Autodesk Fusion 360 part; units mm, degrees
(part 5 of 7)
  spline S12 degree 5 poles (-11.7607, -34.2754) (-11.7671, -34.2886) (-11.7798, -34.3151) (-11.7979, -34.3554) (-11.8201, -34.4098) (-11.8455, -34.4789) (-11.8692, -34.5488) (-11.8917, -34.619) (-11.9136, -34.6896) (-11.9352, -34.7603) (-11.9563, -34.8311) (-11.9769, -34.9022) (-11.9967, -34.9736) (-12.0157, -35.0453) (-12.0338, -35.1173) (-12.0511, -35.1896) (-12.0678, -35.2622) (-12.0838, -35.3349) (-12.0994, -35.4079) (-12.1145, -35.481) (-12.1291, -35.5542) (-12.1432, -35.6277) (-12.1568, -35.7013) (-12.1698, -35.775) (-12.1823, -35.849) (-12.1944, -35.9231) (-12.2059, -35.9974) (-12.2169, -36.0718) (-12.2275, -36.1463) (-12.2377, -36.221) (-12.2474, -36.2958) (-12.2567, -36.3708) (-12.2656, -36.4458) (-12.274, -36.521) (-12.282, -36.5963) (-12.2896, -36.6717) (-12.2968, -36.7473) (-12.3036, -36.8229) (-12.3099, -36.8987) (-12.3159, -36.9745) (-12.3215, -37.0505) (-12.3267, -37.1265) (-12.3315, -37.2027) (-12.336, -37.2789) (-12.34, -37.3553) (-12.3437, -37.4317) (-12.347, -37.5082) (-12.35, -37.5848) (-12.3525, -37.6615) (-12.3548, -37.7383) (-12.3566, -37.8151) (-12.3581, -37.892) (-12.3593, -37.969) (-12.3601, -38.0461) (-12.3606, -38.1232) (-12.3607, -38.2004) (-12.3605, -38.2777) (-12.3599, -38.3551) (-12.359, -38.4325) (-12.3578, -38.51) (-12.3562, -38.5875) (-12.3543, -38.6651) (-12.3521, -38.7428) (-12.3495, -38.8205) (-12.3467, -38.8983) (-12.3435, -38.9761) (-12.34, -39.054) (-12.3361, -39.132) (-12.332, -39.21) (-12.3275, -39.288) (-12.3227, -39.3661) (-12.3186, -39.4286) (-12.3154, -39.4756) (-12.3132, -39.5068) (-12.3121, -39.5225) knots 0 0 0 0 0 0 0.01428571 0.02857143 0.04285714 0.05714286 0.07142857 0.08571429 0.1 0.11428571 0.12857143 0.14285714 0.15714286 0.17142857 0.18571429 0.2 0.21428571 0.22857143 0.24285714 0.25714286 0.27142857 0.28571429 0.3 0.31428571 0.32857143 0.34285714 0.35714286 0.37142857 0.38571429 0.4 0.41428571 0.42857143 0.44285714 0.45714286 0.47142857 0.48571429 0.5 0.51428571 0.52857143 0.54285714 0.55714286 0.57142857 0.58571429 0.6 0.61428571 0.62857143 0.64285714 0.65714286 0.67142857 0.68571429 0.7 0.71428571 0.72857143 0.74285714 0.75714286 0.77142857 0.78571429 0.8 0.81428571 0.82857143 0.84285714 0.85714286 0.87142857 0.88571429 0.9 0.91428571 0.92857143 0.94285714 0.95714286 0.97142857 0.98571429 1 1 1 1 1 1
  arc A27 (-12.3121, -39.5225) -> (-10.5685, -40.2447) centre (5.08, 0) ccw
  spline S13 degree 5 poles (-10.5685, -40.2447) (-10.5567, -40.2344) (-10.533, -40.2139) (-10.4976, -40.183) (-10.4505, -40.1416) (-10.3919, -40.0898) (-10.3335, -40.0378) (-10.2754, -39.9855) (-10.2176, -39.9331) (-10.16, -39.8806) (-10.1027, -39.8278) (-10.0457, -39.7748) (-9.9889, -39.7217) (-9.9325, -39.6683) (-9.8762, -39.6148) (-9.8203, -39.561) (-9.7646, -39.5071) (-9.7093, -39.453) (-9.6542, -39.3987) (-9.5994, -39.3442) (-9.5448, -39.2895) (-9.4906, -39.2347) (-9.4367, -39.1796) (-9.3831, -39.1243) (-9.3298, -39.0689) (-9.2767, -39.0132) (-9.224, -38.9574) (-9.1716, -38.9013) (-9.1196, -38.8451) (-9.0678, -38.7886) (-9.0164, -38.732) (-8.9652, -38.6751) (-8.9145, -38.6181) (-8.864, -38.5608) (-8.8139, -38.5034) (-8.7642, -38.4457) (-8.7148, -38.3878) (-8.6657, -38.3298) (-8.617, -38.2715) (-8.5687, -38.213) (-8.5207, -38.1543) (-8.4731, -38.0954) (-8.4259, -38.0363) (-8.3791, -37.9769) (-8.3327, -37.9174) (-8.2867, -37.8576) (-8.2411, -37.7976) (-8.1958, -37.7374) (-8.151, -37.6769) (-8.1067, -37.6163) (-8.0627, -37.5554) (-8.0193, -37.4942) (-7.9764, -37.4329) (-7.9339, -37.3712) (-7.892, -37.3093) (-7.8505, -37.2472) (-7.8095, -37.1848) (-7.7689, -37.1222) (-7.7288, -37.0594) (-7.6893, -36.9964) (-7.6504, -36.933) (-7.6122, -36.8692) (-7.575, -36.8051) (-7.5385, -36.7406) (-7.5028, -36.6758) (-7.4677, -36.6108) (-7.4329, -36.5456) (-7.3986, -36.4802) (-7.3648, -36.4145) (-7.3321, -36.3484) (-7.3012, -36.2816) (-7.2785, -36.2274) (-7.2628, -36.1862) (-7.253, -36.1584) (-7.2482, -36.1445) knots -1 -1 -1 -1 -1 -1 -0.98571429 -0.97142857 -0.95714286 -0.94285714 -0.92857143 -0.91428571 -0.9 -0.88571429 -0.87142857 -0.85714286 -0.84285714 -0.82857143 -0.81428571 -0.8 -0.78571429 -0.77142857 -0.75714286 -0.74285714 -0.72857143 -0.71428571 -0.7 -0.68571429 -0.67142857 -0.65714286 -0.64285714 -0.62857143 -0.61428571 -0.6 -0.58571429 -0.57142857 -0.55714286 -0.54285714 -0.52857143 -0.51428571 -0.5 -0.48571429 -0.47142857 -0.45714286 -0.44285714 -0.42857143 -0.41428571 -0.4 -0.38571429 -0.37142857 -0.35714286 -0.34285714 -0.32857143 -0.31428571 -0.3 -0.28571429 -0.27142857 -0.25714286 -0.24285714 -0.22857143 -0.21428571 -0.2 -0.18571429 -0.17142857 -0.15714286 -0.14285714 -0.12857143 -0.11428571 -0.1 -0.08571429 -0.07142857 -0.05714286 -0.04285714 -0.02857143 -0.01428571 0 0 0 0 0 0
  line L13 (-7.2482, -36.1445) -> (-7.1541, -35.8689)
  arc A28 (-6.7537, -35.6701) -> (-7.1541, -35.8689) centre (-6.8537, -35.9715) ccw
  arc A29 (-6.7537, -35.6701) -> (-4.8979, -36.2331) centre (5.08, 0) ccw
  arc A30 (-4.6754, -36.6208) -> (-4.8979, -36.2331) centre (-4.9822, -36.5392) ccw
  line L14 (-4.6754, -36.6208) -> (-4.7503, -36.9022)
  spline S14 degree 5 poles (-4.7503, -36.9022) (-4.7541, -36.9164) (-4.7613, -36.945) (-4.7712, -36.988) (-4.7824, -37.0457) (-4.7938, -37.1184) (-4.8034, -37.1915) (-4.8117, -37.2649) (-4.8195, -37.3383) (-4.8269, -37.4119) (-4.8338, -37.4855) (-4.8401, -37.5592) (-4.8456, -37.6331) (-4.8502, -37.7071) (-4.854, -37.7813) (-4.8568, -37.8556) (-4.859, -37.93) (-4.8605, -38.0045) (-4.8616, -38.0791) (-4.8621, -38.1537) (-4.8621, -38.2284) (-4.8616, -38.3032) (-4.8606, -38.378) (-4.859, -38.4529) (-4.8569, -38.5279) (-4.8542, -38.6029) (-4.851, -38.678) (-4.8473, -38.7531) (-4.8432, -38.8283) (-4.8386, -38.9036) (-4.8335, -38.9788) (-4.828, -39.0541) (-4.8221, -39.1295) (-4.8157, -39.2049) (-4.8088, -39.2803) (-4.8016, -39.3558) (-4.7939, -39.4312) (-4.7857, -39.5068) (-4.7772, -39.5823) (-4.7683, -39.6579) (-4.7589, -39.7334) (-4.7492, -39.809) (-4.7391, -39.8847) (-4.7286, -39.9603) (-4.7176, -40.036) (-4.7063, -40.1116) (-4.6947, -40.1873) (-4.6826, -40.263) (-4.6702, -40.3388) (-4.6574, -40.4145) (-4.6442, -40.4902) (-4.6307, -40.5659) (-4.6168, -40.6417) (-4.6026, -40.7174) (-4.588, -40.7932) (-4.573, -40.8689) (-4.5577, -40.9447) (-4.5421, -41.0205) (-4.5261, -41.0962) (-4.5098, -41.172) (-4.4931, -41.2477) (-4.4761, -41.3235) (-4.4588, -41.3992) (-4.4411, -41.4749) (-4.4231, -41.5507) (-4.4048, -41.6264) (-4.3862, -41.7021) (-4.3672, -41.7778) (-4.3479, -41.8535) (-4.3283, -41.9292) (-4.3084, -42.0048) (-4.2922, -42.0653) (-4.2799, -42.1107) (-4.2716, -42.141) (-4.2675, -42.1561) knots 0 0 0 0 0 0 0.01428571 0.02857143 0.04285714 0.05714286 0.07142857 0.08571429 0.1 0.11428571 0.12857143 0.14285714 0.15714286 0.17142857 0.18571429 0.2 0.21428571 0.22857143 0.24285714 0.25714286 0.27142857 0.28571429 0.3 0.31428571 0.32857143 0.34285714 0.35714286 0.37142857 0.38571429 0.4 0.41428571 0.42857143 0.44285714 0.45714286 0.47142857 0.48571429 0.5 0.51428571 0.52857143 0.54285714 0.55714286 0.57142857 0.58571429 0.6 0.61428571 0.62857143 0.64285714 0.65714286 0.67142857 0.68571429 0.7 0.71428571 0.72857143 0.74285714 0.75714286 0.77142857 0.78571429 0.8 0.81428571 0.82857143 0.84285714 0.85714286 0.87142857 0.88571429 0.9 0.91428571 0.92857143 0.94285714 0.95714286 0.97142857 0.98571429 1 1 1 1 1 1
  arc A31 (-4.2675, -42.1561) -> (-2.4165, -42.5243) centre (5.08, 0) ccw
  spline S15 degree 5 poles (-2.4165, -42.5243) (-2.4069, -42.5119) (-2.3877, -42.4871) (-2.3589, -42.4499) (-2.3208, -42.4002) (-2.2735, -42.3379) (-2.2264, -42.2755) (-2.1796, -42.2129) (-2.1331, -42.1503) (-2.0869, -42.0874) (-2.041, -42.0245) (-1.9954, -41.9614) (-1.9501, -41.8982) (-1.9051, -41.8349) (-1.8604, -41.7714) (-1.816, -41.7078) (-1.7719, -41.6441) (-1.7282, -41.5802) (-1.6847, -41.5162) (-1.6416, -41.452) (-1.5988, -41.3878) (-1.5564, -41.3234) (-1.5142, -41.2588) (-1.4724, -41.1942) (-1.4309, -41.1294) (-1.3898, -41.0644) (-1.349, -40.9994) (-1.3085, -40.9342) (-1.2684, -40.8689) (-1.2287, -40.8034) (-1.1893, -40.7378) (-1.1502, -40.6721) (-1.1116, -40.6062) (-1.0733, -40.5402) (-1.0353, -40.4741) (-0.9978, -40.4079) (-0.9606, -40.3415) (-0.9238, -40.2749) (-0.8874, -40.2083) (-0.8514, -40.1415) (-0.8158, -40.0746) (-0.7806, -40.0075) (-0.7459, -39.9403) (-0.7116, -39.873) (-0.6777, -39.8055) (-0.6442, -39.7379) (-0.6112, -39.6701) (-0.5786, -39.6023) (-0.5464, -39.5342) (-0.5147, -39.4661) (-0.4835, -39.3978) (-0.4528, -39.3293) (-0.4227, -39.2608) (-0.3931, -39.192) (-0.364, -39.1231) (-0.3355, -39.0541) (-0.3074, -38.9849) (-0.2798, -38.9156) (-0.2528, -38.8462) (-0.2263, -38.7766) (-0.2005, -38.7069) (-0.1755, -38.6369) (-0.1515, -38.5668) (-0.1283, -38.4964) (-0.106, -38.4259) (-0.0842, -38.3553) (-0.0628, -38.2845) (-0.0419, -38.2136) (-0.0216, -38.1427) (-0.0024, -38.0715) (0.0149, -37.9999) (0.0266, -37.9423) (0.0339, -37.8988) (0.0382, -37.8697) (0.0401, -37.8551) knots -1 -1 -1 -1 -1 -1 -0.98571429 -0.97142857 -0.95714286 -0.94285714 -0.92857143 -0.91428571 -0.9 -0.88571429 -0.87142857 -0.85714286 -0.84285714 -0.82857143 -0.81428571 -0.8 -0.78571429 -0.77142857 -0.75714286 -0.74285714 -0.72857143 -0.71428571 -0.7 -0.68571429 -0.67142857 -0.65714286 -0.64285714 -0.62857143 -0.61428571 -0.6 -0.58571429 -0.57142857 -0.55714286 -0.54285714 -0.52857143 -0.51428571 -0.5 -0.48571429 -0.47142857 -0.45714286 -0.44285714 -0.42857143 -0.41428571 -0.4 -0.38571429 -0.37142857 -0.35714286 -0.34285714 -0.32857143 -0.31428571 -0.3 -0.28571429 -0.27142857 -0.25714286 -0.24285714 -0.22857143 -0.21428571 -0.2 -0.18571429 -0.17142857 -0.15714286 -0.14285714 -0.12857143 -0.11428571 -0.1 -0.08571429 -0.07142857 -0.05714286 -0.04285714 -0.02857143 -0.01428571 0 0 0 0 0 0
  line L15 (0.0401, -37.8551) -> (0.0786, -37.5665)
  arc A32 (0.4326, -37.2934) -> (0.0786, -37.5665) centre (0.3933, -37.6084) ccw
  arc A33 (0.4326, -37.2934) -> (2.3625, -37.4835) centre (5.08, 0) ccw
  arc A34 (2.6564, -37.8204) -> (2.3625, -37.4835) centre (2.3396, -37.8001) ccw
  line L16 (2.6564, -37.8204) -> (2.6379, -38.1109)
  spline S16 degree 5 poles (2.6379, -38.1109) (2.6369, -38.1256) (2.6354, -38.155) (2.6341, -38.1991) (2.6344, -38.2579) (2.6374, -38.3315) (2.6423, -38.405) (2.6483, -38.4786) (2.6551, -38.5522) (2.6622, -38.6257) (2.6698, -38.6993) (2.678, -38.7728) (2.687, -38.8464) (2.6969, -38.9198) (2.7077, -38.9933) (2.7194, -39.0668) (2.7318, -39.1402) (2.7448, -39.2135) (2.7583, -39.2869) (2.7724, -39.3602) (2.7869, -39.4335) (2.802, -39.5067) (2.8176, -39.5799) (2.8337, -39.653) (2.8505, -39.7262) (2.8678, -39.7992) (2.8855, -39.8723) (2.9038, -39.9452) (2.9225, -40.0182) (2.9417, -40.0911) (2.9614, -40.1639) (2.9814, -40.2367) (3.002, -40.3094) (3.023, -40.3821) (3.0444, -40.4548) (3.0662, -40.5273) (3.0885, -40.5999) (3.1112, -40.6724) (3.1343, -40.7448) (3.1578, -40.8171) (3.1817, -40.8895) (3.206, -40.9617) (3.2307, -41.0339) (3.2558, -41.106) (3.2813, -41.1781) (3.3071, -41.2501) (3.3333, -41.3221) (3.3599, -41.394) (3.3869, -41.4658) (3.4142, -41.5376) (3.4419, -41.6093) (3.4699, -41.6809) (3.4983, -41.7525) (3.527, -41.824) (3.5561, -41.8955) (3.5856, -41.9669) (3.6154, -42.0382) (3.6455, -42.1094) (3.6759, -42.1806) (3.7067, -42.2517) (3.7378, -42.3228) (3.7693, -42.3938) (3.8011, -42.4647) (3.8332, -42.5355) (3.8656, -42.6063) (3.8983, -42.6769) (3.9314, -42.7476) (3.9648, -42.8181) (3.9985, -42.8886) (4.0325, -42.959) (4.0668, -43.0293) (4.0944, -43.0855) (4.1154, -43.1276) (4.1294, -43.1557) (4.1364, -43.1697) knots 0 0 0 0 0 0 0.01428571 0.02857143 0.04285714 0.05714286 0.07142857 0.08571429 0.1 0.11428571 0.12857143 0.14285714 0.15714286 0.17142857 0.18571429 0.2 0.21428571 0.22857143 0.24285714 0.25714286 0.27142857 0.28571429 0.3 0.31428571 0.32857143 0.34285714 0.35714286 0.37142857 0.38571429 0.4 0.41428571 0.42857143 0.44285714 0.45714286 0.47142857 0.48571429 0.5 0.51428571 0.52857143 0.54285714 0.55714286 0.57142857 0.58571429 0.6 0.61428571 0.62857143 0.64285714 0.65714286 0.67142857 0.68571429 0.7 0.71428571 0.72857143 0.74285714 0.75714286 0.77142857 0.78571429 0.8 0.81428571 0.82857143 0.84285714 0.85714286 0.87142857 0.88571429 0.9 0.91428571 0.92857143 0.94285714 0.95714286 0.97142857 0.98571429 1 1 1 1 1 1
  arc A35 (4.1364, -43.1697) -> (6.0236, -43.1697) centre (5.08, 0) ccw
  spline S17 degree 5 poles (6.0236, -43.1697) (6.0306, -43.1557) (6.0446, -43.1276) (6.0656, -43.0855) (6.0932, -43.0293) (6.1275, -42.959) (6.1615, -42.8886) (6.1952, -42.8181) (6.2286, -42.7476) (6.2617, -42.6769) (6.2944, -42.6063) (6.3268, -42.5355) (6.3589, -42.4647) (6.3907, -42.3938) (6.4222, -42.3228) (6.4533, -42.2517) (6.4841, -42.1806) (6.5145, -42.1094) (6.5446, -42.0382) (6.5744, -41.9669) (6.6039, -41.8955) (6.633, -41.824) (6.6617, -41.7525) (6.6901, -41.6809) (6.7181, -41.6093) (6.7458, -41.5376) (6.7731, -41.4658) (6.8001, -41.394) (6.8267, -41.3221) (6.8529, -41.2501) (6.8787, -41.1781) (6.9042, -41.106) (6.9293, -41.0339) (6.954, -40.9617) (6.9783, -40.8895) (7.0022, -40.8171) (7.0257, -40.7448) (7.0488, -40.6724) (7.0715, -40.5999) (7.0938, -40.5273) (7.1156, -40.4548) (7.137, -40.3821) (7.158, -40.3094) (7.1786, -40.2367) (7.1986, -40.1639) (7.2183, -40.0911) (7.2375, -40.0182) (7.2562, -39.9452) (7.2745, -39.8723) (7.2922, -39.7992) (7.3095, -39.7262) (7.3263, -39.653) (7.3424, -39.5799) (7.358, -39.5067) (7.3731, -39.4335) (7.3876, -39.3602) (7.4017, -39.2869) (7.4152, -39.2135) (7.4282, -39.1402) (7.4406, -39.0668) (7.4523, -38.9933) (7.4631, -38.9198) (7.473, -38.8464) (7.482, -38.7728) (7.4902, -38.6993) (7.4978, -38.6257) (7.5049, -38.5522) (7.5117, -38.4786) (7.5177, -38.405) (7.5226, -38.3315) (7.5256, -38.2579) (7.5259, -38.1991) (7.5246, -38.155) (7.5231, -38.1256) (7.5221, -38.1109) knots -1 -1 -1 -1 -1 -1 -0.98571429 -0.97142857 -0.95714286 -0.94285714 -0.92857143 -0.91428571 -0.9 -0.88571429 -0.87142857 -0.85714286 -0.84285714 -0.82857143 -0.81428571 -0.8 -0.78571429 -0.77142857 -0.75714286 -0.74285714 -0.72857143 -0.71428571 -0.7 -0.68571429 -0.67142857 -0.65714286 -0.64285714 -0.62857143 -0.61428571 -0.6 -0.58571429 -0.57142857 -0.55714286 -0.54285714 -0.52857143 -0.51428571 -0.5 -0.48571429 -0.47142857 -0.45714286 -0.44285714 -0.42857143 -0.41428571 -0.4 -0.38571429 -0.37142857 -0.35714286 -0.34285714 -0.32857143 -0.31428571 -0.3 -0.28571429 -0.27142857 -0.25714286 -0.24285714 -0.22857143 -0.21428571 -0.2 -0.18571429 -0.17142857 -0.15714286 -0.14285714 -0.12857143 -0.11428571 -0.1 -0.08571429 -0.07142857 -0.05714286 -0.04285714 -0.02857143 -0.01428571 0 0 0 0 0 0
  line L17 (7.5221, -38.1109) -> (7.5036, -37.8204)
  arc A36 (7.7975, -37.4835) -> (7.5036, -37.8204) centre (7.8204, -37.8001) ccw
  arc A37 (7.7975, -37.4835) -> (9.7274, -37.2934) centre (5.08, 0) ccw
  arc A38 (10.0814, -37.5665) -> (9.7274, -37.2934) centre (9.7667, -37.6084) ccw
  line L18 (10.0814, -37.5665) -> (10.1199, -37.8551)
  spline S18 degree 5 poles (10.1199, -37.8551) (10.1218, -37.8697) (10.1261, -37.8988) (10.1334, -37.9423) (10.1451, -37.9999) (10.1624, -38.0715) (10.1816, -38.1427) (10.2019, -38.2136) (10.2228, -38.2845) (10.2442, -38.3553) (10.266, -38.4259) (10.2883, -38.4964) (10.3115, -38.5668) (10.3355, -38.6369) (10.3605, -38.7069) (10.3863, -38.7766) (10.4128, -38.8462) (10.4398, -38.9156) (10.4674, -38.9849) (10.4955, -39.0541) (10.524, -39.1231) (10.5531, -39.192) (10.5827, -39.2608) (10.6128, -39.3293) (10.6435, -39.3978) (10.6747, -39.4661) (10.7064, -39.5342) (10.7386, -39.6023) (10.7712, -39.6701) (10.8042, -39.7379) (10.8377, -39.8055) (10.8716, -39.873) (10.9059, -39.9403) (10.9406, -40.0075) (10.9758, -40.0746) (11.0114, -40.1415) (11.0474, -40.2083) (11.0838, -40.2749) (11.1206, -40.3415) (11.1578, -40.4079) (11.1953, -40.4741) (11.2333, -40.5402) (11.2716, -40.6062) (11.3102, -40.6721) (11.3493, -40.7378) (11.3887, -40.8034) (11.4284, -40.8689) (11.4685, -40.9342) (11.509, -40.9994) (11.5498, -41.0644) (11.5909, -41.1294) (11.6324, -41.1942) (11.6742, -41.2588) (11.7164, -41.3234) (11.7588, -41.3878) (11.8016, -41.452) (11.8447, -41.5162) (11.8882, -41.5802) (11.9319, -41.6441) (11.976, -41.7078) (12.0204, -41.7714) (12.0651, -41.8349) (12.1101, -41.8982) (12.1554, -41.9614) (12.201, -42.0245) (12.2469, -42.0874) (12.2931, -42.1503) (12.3396, -42.2129) (12.3864, -42.2755) (12.4335, -42.3379) (12.4808, -42.4002) (12.5189, -42.4499) (12.5477, -42.4871) (12.5669, -42.5119) (12.5765, -42.5243) knots 0 0 0 0 0 0 0.01428571 0.02857143 0.04285714 0.05714286 0.07142857 0.08571429 0.1 0.11428571 0.12857143 0.14285714 0.15714286 0.17142857 0.18571429 0.2 0.21428571 0.22857143 0.24285714 0.25714286 0.27142857 0.28571429 0.3 0.31428571 0.32857143 0.34285714 0.35714286 0.37142857 0.38571429 0.4 0.41428571 0.42857143 0.44285714 0.45714286 0.47142857 0.48571429 0.5 0.51428571 0.52857143 0.54285714 0.55714286 0.57142857 0.58571429 0.6 0.61428571 0.62857143 0.64285714 0.65714286 0.67142857 0.68571429 0.7 0.71428571 0.72857143 0.74285714 0.75714286 0.77142857 0.78571429 0.8 0.81428571 0.82857143 0.84285714 0.85714286 0.87142857 0.88571429 0.9 0.91428571 0.92857143 0.94285714 0.95714286 0.97142857 0.98571429 1 1 1 1 1 1
  arc A39 (12.5765, -42.5243) -> (14.4275, -42.1561) centre (5.08, 0) ccw
  spline S19 degree 5 poles (14.4275, -42.1561) (14.4316, -42.141) (14.4399, -42.1107) (14.4522, -42.0653) (14.4684, -42.0048) (14.4883, -41.9292) (14.5079, -41.8535) (14.5272, -41.7778) (14.5462, -41.7021) (14.5648, -41.6264) (14.5831, -41.5507) (14.6011, -41.4749) (14.6188, -41.3992) (14.6361, -41.3235) (14.6531, -41.2477) (14.6698, -41.172) (14.6861, -41.0962) (14.7021, -41.0205) (14.7177, -40.9447) (14.733, -40.8689) (14.748, -40.7932) (14.7626, -40.7174) (14.7768, -40.6417) (14.7907, -40.5659) (14.8042, -40.4902) (14.8174, -40.4145) (14.8302, -40.3388) (14.8426, -40.263) (14.8547, -40.1873) (14.8663, -40.1116) (14.8776, -40.036) (14.8886, -39.9603) (14.8991, -39.8847) (14.9092, -39.809) (14.9189, -39.7334) (14.9283, -39.6579) (14.9372, -39.5823) (14.9457, -39.5068) (14.9539, -39.4312) (14.9616, -39.3558) (14.9688, -39.2803) (14.9757, -39.2049) (14.9821, -39.1295) (14.988, -39.0541) (14.9935, -38.9788) (14.9986, -38.9036) (15.0032, -38.8283) (15.0073, -38.7531) (15.011, -38.678) (15.0142, -38.6029) (15.0169, -38.5279) (15.019, -38.4529) (15.0206, -38.378) (15.0216, -38.3032) (15.0221, -38.2284) (15.0221, -38.1537) (15.0216, -38.0791) (15.0205, -38.0045) (15.019, -37.93) (15.0168, -37.8556) (15.014, -37.7813) (15.0102, -37.7071) (15.0056, -37.6331) (15.0001, -37.5592) (14.9938, -37.4855) (14.9869, -37.4119) (14.9795, -37.3383) (14.9717, -37.2649) (14.9634, -37.1915) (14.9538, -37.1184) (14.9424, -37.0457) (14.9312, -36.988) (14.9213, -36.945) (14.9141, -36.9164) (14.9103, -36.9022) knots -1 -1 -1 -1 -1 -1 -0.98571429 -0.97142857 -0.95714286 -0.94285714 -0.92857143 -0.91428571 -0.9 -0.88571429 -0.87142857 -0.85714286 -0.84285714 -0.82857143 -0.81428571 -0.8 -0.78571429 -0.77142857 -0.75714286 -0.74285714 -0.72857143 -0.71428571 -0.7 -0.68571429 -0.67142857 -0.65714286 -0.64285714 -0.62857143 -0.61428571 -0.6 -0.58571429 -0.57142857 -0.55714286 -0.54285714 -0.52857143 -0.51428571 -0.5 -0.48571429 -0.47142857 -0.45714286 -0.44285714 -0.42857143 -0.41428571 -0.4 -0.38571429 -0.37142857 -0.35714286 -0.34285714 -0.32857143 -0.31428571 -0.3 -0.28571429 -0.27142857 -0.25714286 -0.24285714 -0.22857143 -0.21428571 -0.2 -0.18571429 -0.17142857 -0.15714286 -0.14285714 -0.12857143 -0.11428571 -0.1 -0.08571429 -0.07142857 -0.05714286 -0.04285714 -0.02857143 -0.01428571 0 0 0 0 0 0
  line L19 (14.9103, -36.9022) -> (14.8354, -36.6208)
  arc A40 (15.0579, -36.2331) -> (14.8354, -36.6208) centre (15.1422, -36.5392) ccw
  arc A41 (15.0579, -36.2331) -> (16.9137, -35.6701) centre (5.08, 0) ccw
  arc A42 (17.3141, -35.8689) -> (16.9137, -35.6701) centre (17.0137, -35.9715) ccw
  line L20 (17.3141, -35.8689) -> (17.4082, -36.1445)
  spline S20 degree 5 poles (17.4082, -36.1445) (17.413, -36.1584) (17.4228, -36.1862) (17.4385, -36.2274) (17.4612, -36.2816) (17.4921, -36.3484) (17.5248, -36.4145) (17.5586, -36.4802) (17.5929, -36.5456) (17.6277, -36.6108) (17.6628, -36.6758) (17.6985, -36.7406) (17.735, -36.8051) (17.7722, -36.8692) (17.8104, -36.933) (17.8493, -36.9964) (17.8888, -37.0594) (17.9289, -37.1222) (17.9695, -37.1848) (18.0105, -37.2472) (18.052, -37.3093) (18.0939, -37.3712) (18.1364, -37.4329) (18.1793, -37.4942) (18.2227, -37.5554) (18.2667, -37.6163) (18.311, -37.6769) (18.3558, -37.7374) (18.4011, -37.7976) (18.4467, -37.8576) (18.4927, -37.9174) (18.5391, -37.9769) (18.5859, -38.0363) (18.6331, -38.0954) (18.6807, -38.1543) (18.7287, -38.213) (18.777, -38.2715) (18.8257, -38.3298) (18.8748, -38.3878) (18.9242, -38.4457) (18.9739, -38.5034) (19.024, -38.5608) (19.0745, -38.6181) (19.1252, -38.6751) (19.1764, -38.732) (19.2278, -38.7886) (19.2796, -38.8451) (19.3316, -38.9013) (19.384, -38.9574) (19.4367, -39.0132) (19.4898, -39.0689) (19.5431, -39.1243) (19.5967, -39.1796) (19.6506, -39.2347) (19.7048, -39.2895) (19.7594, -39.3442) (19.8142, -39.3987) (19.8693, -39.453) (19.9246, -39.5071) (19.9803, -39.561) (20.0362, -39.6148) (20.0925, -39.6683) (20.1489, -39.7217) (20.2057, -39.7748) (20.2627, -39.8278) (20.32, -39.8806) (20.3776, -39.9331) (20.4354, -39.9855) (20.4935, -40.0378) (20.5519, -40.0898) (20.6105, -40.1416) (20.6576, -40.183) (20.693, -40.2139) (20.7167, -40.2344) (20.7285, -40.2447) knots 0 0 0 0 0 0 0.01428571 0.02857143 0.04285714 0.05714286 0.07142857 0.08571429 0.1 0.11428571 0.12857143 0.14285714 0.15714286 0.17142857 0.18571429 0.2 0.21428571 0.22857143 0.24285714 0.25714286 0.27142857 0.28571429 0.3 0.31428571 0.32857143 0.34285714 0.35714286 0.37142857 0.38571429 0.4 0.41428571 0.42857143 0.44285714 0.45714286 0.47142857 0.48571429 0.5 0.51428571 0.52857143 0.54285714 0.55714286 0.57142857 0.58571429 0.6 0.61428571 0.62857143 0.64285714 0.65714286 0.67142857 0.68571429 0.7 0.71428571 0.72857143 0.74285714 0.75714286 0.77142857 0.78571429 0.8 0.81428571 0.82857143 0.84285714 0.85714286 0.87142857 0.88571429 0.9 0.91428571 0.92857143 0.94285714 0.95714286 0.97142857 0.98571429 1 1 1 1 1 1
  arc A43 (20.7285, -40.2447) -> (22.4721, -39.5225) centre (5.08, 0) ccw
  spline S21 degree 5 poles (22.4721, -39.5225) (22.4732, -39.5068) (22.4754, -39.4756) (22.4786, -39.4286) (22.4827, -39.3661) (22.4875, -39.288) (22.492, -39.21) (22.4961, -39.132) (22.5, -39.054) (22.5035, -38.9761) (22.5067, -38.8983) (22.5095, -38.8205) (22.5121, -38.7428) (22.5143, -38.6651) (22.5162, -38.5875) (22.5178, -38.51) (22.519, -38.4325) (22.5199, -38.3551) (22.5205, -38.2777) (22.5207, -38.2004) (22.5206, -38.1232) (22.5201, -38.0461) (22.5193, -37.969) (22.5181, -37.892) (22.5166, -37.8151) (22.5148, -37.7383) (22.5125, -37.6615) (22.51, -37.5848) (22.507, -37.5082) (22.5037, -37.4317) (22.5, -37.3553) (22.496, -37.2789) (22.4915, -37.2027) (22.4867, -37.1265) (22.4815, -37.0505) (22.4759, -36.9745) (22.4699, -36.8987) (22.4636, -36.8229) (22.4568, -36.7473) (22.4496, -36.6717) (22.442, -36.5963) (22.434, -36.521) (22.4256, -36.4458) (22.4167, -36.3708) (22.4074, -36.2958) (22.3977, -36.221) (22.3875, -36.1463) (22.3769, -36.0718) (22.3659, -35.9974) (22.3544, -35.9231) (22.3423, -35.849) (22.3298, -35.775) (22.3168, -35.7013) (22.3032, -35.6277) (22.2891, -35.5542) (22.2745, -35.481) (22.2594, -35.4079) (22.2438, -35.3349) (22.2278, -35.2622) (22.2111, -35.1896) (22.1938, -35.1173) (22.1757, -35.0453) (22.1567, -34.9736) (22.1369, -34.9022) (22.1163, -34.8311) (22.0952, -34.7603) (22.0736, -34.6896) (22.0517, -34.619) (22.0292, -34.5488) (22.0055, -34.4789) (21.9801, -34.4098) (21.9579, -34.3554) (21.9398, -34.3151) (21.9271, -34.2886) (21.9207, -34.2754) knots -1 -1 -1 -1 -1 -1 -0.98571429 -0.97142857 -0.95714286 -0.94285714 -0.92857143 -0.91428571 -0.9 -0.88571429 -0.87142857 -0.85714286 -0.84285714 -0.82857143 -0.81428571 -0.8 -0.78571429 -0.77142857 -0.75714286 -0.74285714 -0.72857143 -0.71428571 -0.7 -0.68571429 -0.67142857 -0.65714286 -0.64285714 -0.62857143 -0.61428571 -0.6 -0.58571429 -0.57142857 -0.55714286 -0.54285714 -0.52857143 -0.51428571 -0.5 -0.48571429 -0.47142857 -0.45714286 -0.44285714 -0.42857143 -0.41428571 -0.4 -0.38571429 -0.37142857 -0.35714286 -0.34285714 -0.32857143 -0.31428571 -0.3 -0.28571429 -0.27142857 -0.25714286 -0.24285714 -0.22857143 -0.21428571 -0.2 -0.18571429 -0.17142857 -0.15714286 -0.14285714 -0.12857143 -0.11428571 -0.1 -0.08571429 -0.07142857 -0.05714286 -0.04285714 -0.02857143 -0.01428571 0 0 0 0 0 0
  line L21 (21.9207, -34.2754) -> (21.7923, -34.014)
  arc A44 (21.9349, -33.5903) -> (21.7923, -34.014) centre (22.0773, -33.8741) ccw
  arc A45 (21.9349, -33.5903) -> (23.6452, -32.6761) centre (5.08, 0) ccw
  arc A46 (24.0768, -32.7929) -> (23.6452, -32.6761) centre (23.8021, -32.9522) ccw
  line L22 (24.0768, -32.7929) -> (24.2228, -33.0449)
  spline S22 degree 5 poles (24.2228, -33.0449) (24.2301, -33.0576) (24.2452, -33.0829) (24.2686, -33.1203) (24.3015, -33.169) (24.3449, -33.2285) (24.3898, -33.287) (24.4357, -33.3448) (24.4822, -33.4022) (24.529, -33.4594) (24.5762, -33.5163) (24.6238, -33.5729) (24.6721, -33.6291) (24.7212, -33.6847) (24.771, -33.7397) (24.8215, -33.7943) (24.8726, -33.8485) (24.9242, -33.9022) (24.9762, -33.9557) (25.0286, -34.0089) (25.0814, -34.0617) (25.1346, -34.1142) (25.1883, -34.1664) (25.2424, -34.2183) (25.2969, -34.2698) (25.3519, -34.3209) (25.4072, -34.3717) (25.463, -34.4223) (25.519, -34.4725) (25.5755, -34.5225) (25.6323, -34.5721) (25.6894, -34.6215) (25.7469, -34.6706) (25.8047, -34.7193) (25.8629, -34.7678) (25.9214, -34.816) (25.9802, -34.864) (26.0394, -34.9116) (26.0988, -34.959) (26.1585, -35.0061) (26.2186, -35.053) (26.2789, -35.0995) (26.3396, -35.1459) (26.4005, -35.1919) (26.4617, -35.2377) (26.5232, -35.2832) (26.585, -35.3285) (26.6471, -35.3735) (26.7094, -35.4182) (26.772, -35.4627) (26.8348, -35.507) (26.898, -35.551) (26.9613, -35.5947) (27.025, -35.6382) (27.0888, -35.6814) (27.153, -35.7244) (27.2174, -35.7672) (27.282, -35.8097) (27.3469, -35.852) (27.412, -35.894) (27.4773, -35.9358) (27.5429, -35.9773) (27.6087, -36.0186) (27.6748, -36.0597) (27.741, -36.1005) (27.8075, -36.1411) (27.8742, -36.1814) (27.9412, -36.2215) (28.0083, -36.2614) (28.0757, -36.3011) (28.1433, -36.3405) (28.1976, -36.3718) (28.2383, -36.3952) (28.2656, -36.4108) (28.2792, -36.4185) knots 0 0 0 0 0 0 0.01428571 0.02857143 0.04285714 0.05714286 0.07142857 0.08571429 0.1 0.11428571 0.12857143 0.14285714 0.15714286 0.17142857 0.18571429 0.2 0.21428571 0.22857143 0.24285714 0.25714286 0.27142857 0.28571429 0.3 0.31428571 0.32857143 0.34285714 0.35714286 0.37142857 0.38571429 0.4 0.41428571 0.42857143 0.44285714 0.45714286 0.47142857 0.48571429 0.5 0.51428571 0.52857143 0.54285714 0.55714286 0.57142857 0.58571429 0.6 0.61428571 0.62857143 0.64285714 0.65714286 0.67142857 0.68571429 0.7 0.71428571 0.72857143 0.74285714 0.75714286 0.77142857 0.78571429 0.8 0.81428571 0.82857143 0.84285714 0.85714286 0.87142857 0.88571429 0.9 0.91428571 0.92857143 0.94285714 0.95714286 0.97142857 0.98571429 1 1 1 1 1 1
  arc A47 (28.2792, -36.4185) -> (29.8484, -35.37) centre (5.08, 0) ccw
  spline S23 degree 5 poles (29.8484, -35.37) (29.8464, -35.3545) (29.8425, -35.3234) (29.8365, -35.2767) (29.8283, -35.2146) (29.8177, -35.1371) (29.8069, -35.0597) (29.7957, -34.9824) (29.7843, -34.9052) (29.7726, -34.8281) (29.7605, -34.7511) (29.7482, -34.6743) (29.7355, -34.5975) (29.7225, -34.5209) (29.7092, -34.4444) (29.6956, -34.3681) (29.6817, -34.2918) (29.6675, -34.2157) (29.653, -34.1398) (29.6381, -34.0639) (29.6229, -33.9882) (29.6074, -33.9126) (29.5916, -33.8372) (29.5754, -33.7619) (29.5589, -33.6868) (29.5421, -33.6118) (29.525, -33.5369) (29.5075, -33.4622) (29.4896, -33.3877) (29.4715, -33.3133) (29.4529, -33.239) (29.4341, -33.1649) (29.4148, -33.091) (29.3953, -33.0173) (29.3753, -32.9437) (29.355, -32.8703) (29.3344, -32.7971) (29.3133, -32.724) (29.2919, -32.6511) (29.2702, -32.5785) (29.248, -32.506) (29.2255, -32.4337) (29.2025, -32.3616) (29.1792, -32.2897) (29.1554, -32.218) (29.1313, -32.1465) (29.1068, -32.0753) (29.0818, -32.0042) (29.0565, -31.9334) (29.0307, -31.8628) (29.0044, -31.7924) (28.9777, -31.7224) (28.9506, -31.6525) (28.9229, -31.583) (28.8947, -31.5137) (28.8661, -31.4447) (28.837, -31.376) (28.8075, -31.3075) (28.7776, -31.2392) (28.7471, -31.1713) (28.716, -31.1038) (28.6842, -31.0367) (28.6516, -30.9701) (28.6182, -30.9039) (28.5842, -30.8382) (28.5496, -30.7729) (28.5147, -30.7077) (28.4794, -30.6428) (28.4436, -30.5783) (28.4068, -30.5144) (28.3684, -30.4516) (28.336, -30.4026) (28.3104, -30.3666) (28.2928, -30.343) (28.2839, -30.3313) knots -1 -1 -1 -1 -1 -1 -0.98571429 -0.97142857 -0.95714286 -0.94285714 -0.92857143 -0.91428571 -0.9 -0.88571429 -0.87142857 -0.85714286 -0.84285714 -0.82857143 -0.81428571 -0.8 -0.78571429 -0.77142857 -0.75714286 -0.74285714 -0.72857143 -0.71428571 -0.7 -0.68571429 -0.67142857 -0.65714286 -0.64285714 -0.62857143 -0.61428571 -0.6 -0.58571429 -0.57142857 -0.55714286 -0.54285714 -0.52857143 -0.51428571 -0.5 -0.48571429 -0.47142857 -0.45714286 -0.44285714 -0.42857143 -0.41428571 -0.4 -0.38571429 -0.37142857 -0.35714286 -0.34285714 -0.32857143 -0.31428571 -0.3 -0.28571429 -0.27142857 -0.25714286 -0.24285714 -0.22857143 -0.21428571 -0.2 -0.18571429 -0.17142857 -0.15714286 -0.14285714 -0.12857143 -0.11428571 -0.1 -0.08571429 -0.07142857 -0.05714286 -0.04285714 -0.02857143 -0.01428571 0 0 0 0 0 0
  line L23 (28.2839, -30.3313) -> (28.107, -30.1)
  arc A48 (28.1642, -29.6566) -> (28.107, -30.1) centre (28.3592, -29.9072) ccw
  arc A49 (28.1642, -29.6566) -> (29.6633, -28.4263) centre (5.08, 0) ccw
  arc A50 (30.1093, -28.4568) -> (29.6633, -28.4263) centre (29.871, -28.6665) ccw
  line L24 (30.1093, -28.4568) -> (30.3017, -28.6753)
  spline S24 degree 5 poles (30.3017, -28.6753) (30.3114, -28.6864) (30.3311, -28.7083) (30.3614, -28.7404) (30.4031, -28.7818) (30.4572, -28.8317) (30.5127, -28.8802) (30.569, -28.9279) (30.6258, -28.9752) (30.6829, -29.0222) (30.7403, -29.0688) (30.798, -29.115) (30.8564, -29.1607) (30.9154, -29.2056) (30.975, -29.2499) (31.0351, -29.2936) (31.0958, -29.3367) (31.1569, -29.3794) (31.2184, -29.4217) (31.2801, -29.4636) (31.3422, -29.5051) (31.4046, -29.5463) (31.4674, -29.587) (31.5306, -29.6273) (31.5941, -29.6671) (31.658, -29.7066) (31.7222, -29.7457) (31.7868, -29.7843) (31.8516, -29.8227) (31.9167, -29.8606) (31.9821, -29.8983) (32.0477, -29.9355) (32.1137, -29.9725) (32.1799, -30.009) (32.2464, -30.0452) (32.3132, -30.0811) (32.3803, -30.1166) (32.4475, -30.1518) (32.5151, -30.1867) (32.5829, -30.2213) (32.6509, -30.2555) (32.7192, -30.2894) (32.7877, -30.323) (32.8564, -30.3563) (32.9254, -30.3892) (32.9946, -30.4219) (33.064, -30.4542) (33.1337, -30.4863) (33.2035, -30.518) (33.2736, -30.5494) (33.3439, -30.5806) (33.4144, -30.6114) (33.4851, -30.6419) (33.556, -30.6722) (33.6271, -30.7021) (33.6983, -30.7318) (33.7698, -30.7612) (33.8415, -30.7902) (33.9134, -30.819) (33.9854, -30.8475) (34.0577, -30.8758) (34.1301, -30.9037) (34.2027, -30.9314) (34.2755, -30.9588) (34.3485, -30.9859) (34.4216, -31.0127) (34.4949, -31.0393) (34.5684, -31.0656) (34.642, -31.0916) (34.7158, -31.1173) (34.7898, -31.1428) (34.8491, -31.1629) (34.8937, -31.1779) (34.9235, -31.1879) (34.9383, -31.1928) knots 0 0 0 0 0 0 0.01428571 0.02857143 0.04285714 0.05714286 0.07142857 0.08571429 0.1 0.11428571 0.12857143 0.14285714 0.15714286 0.17142857 0.18571429 0.2 0.21428571 0.22857143 0.24285714 0.25714286 0.27142857 0.28571429 0.3 0.31428571 0.32857143 0.34285714 0.35714286 0.37142857 0.38571429 0.4 0.41428571 0.42857143 0.44285714 0.45714286 0.47142857 0.48571429 0.5 0.51428571 0.52857143 0.54285714 0.55714286 0.57142857 0.58571429 0.6 0.61428571 0.62857143 0.64285714 0.65714286 0.67142857 0.68571429 0.7 0.71428571 0.72857143 0.74285714 0.75714286 0.77142857 0.78571429 0.8 0.81428571 0.82857143 0.84285714 0.85714286 0.87142857 0.88571429 0.9 0.91428571 0.92857143 0.94285714 0.95714286 0.97142857 0.98571429 1 1 1 1 1 1
  arc A51 (34.9383, -31.1928) -> (36.2728, -29.8583) centre (5.08, 0) ccw
  spline S25 degree 5 poles (36.2728, -29.8583) (36.2679, -29.8435) (36.2579, -29.8137) (36.2429, -29.7691) (36.2228, -29.7098) (36.1973, -29.6358) (36.1716, -29.562) (36.1456, -29.4884) (36.1193, -29.4149) (36.0927, -29.3416) (36.0659, -29.2685) (36.0388, -29.1955) (36.0114, -29.1227) (35.9837, -29.0501) (35.9558, -28.9777) (35.9275, -28.9054) (35.899, -28.8334) (35.8702, -28.7615) (35.8412, -28.6898) (35.8118, -28.6183) (35.7821, -28.5471) (35.7522, -28.476) (35.7219, -28.4051) (35.6914, -28.3344) (35.6606, -28.2639) (35.6294, -28.1936) (35.598, -28.1235) (35.5663, -28.0537) (35.5342, -27.984) (35.5019, -27.9146) (35.4692, -27.8454) (35.4363, -27.7764) (35.403, -27.7077) (35.3694, -27.6392) (35.3355, -27.5709) (35.3013, -27.5029) (35.2667, -27.4351) (35.2318, -27.3675) (35.1966, -27.3003) (35.1611, -27.2332) (35.1252, -27.1664) (35.089, -27.0999) (35.0525, -27.0337) (35.0155, -26.9677) (34.9783, -26.9021) (34.9406, -26.8367) (34.9027, -26.7716) (34.8643, -26.7068) (34.8257, -26.6422) (34.7866, -26.578) (34.7471, -26.5141) (34.7073, -26.4506) (34.667, -26.3874) (34.6263, -26.3246) (34.5851, -26.2622) (34.5436, -26.2001) (34.5017, -26.1384) (34.4594, -26.0769) (34.4167, -26.0158) (34.3736, -25.9551) (34.3299, -25.895) (34.2856, -25.8354) (34.2407, -25.7764) (34.195, -25.718) (34.1488, -25.6603) (34.1022, -25.6029) (34.0552, -25.5458) (34.0079, -25.489) (33.9602, -25.4327) (33.9117, -25.3772) (33.8618, -25.3231) (33.8204, -25.2814) (33.7883, -25.2511) (33.7664, -25.2314) (33.7553, -25.2217) knots -1 -1 -1 -1 -1 -1 -0.98571429 -0.97142857 -0.95714286 -0.94285714 -0.92857143 -0.91428571 -0.9 -0.88571429 -0.87142857 -0.85714286 -0.84285714 -0.82857143 -0.81428571 -0.8 -0.78571429 -0.77142857 -0.75714286 -0.74285714 -0.72857143 -0.71428571 -0.7 -0.68571429 -0.67142857 -0.65714286 -0.64285714 -0.62857143 -0.61428571 -0.6 -0.58571429 -0.57142857 -0.55714286 -0.54285714 -0.52857143 -0.51428571 -0.5 -0.48571429 -0.47142857 -0.45714286 -0.44285714 -0.42857143 -0.41428571 -0.4 -0.38571429 -0.37142857 -0.35714286 -0.34285714 -0.32857143 -0.31428571 -0.3 -0.28571429 -0.27142857 -0.25714286 -0.24285714 -0.22857143 -0.21428571 -0.2 -0.18571429 -0.17142857 -0.15714286 -0.14285714 -0.12857143 -0.11428571 -0.1 -0.08571429 -0.07142857 -0.05714286 -0.04285714 -0.02857143 -0.01428571 0 0 0 0 0 0
  line L25 (33.7553, -25.2217) -> (33.5368, -25.0293)
  arc A52 (33.5063, -24.5833) -> (33.5368, -25.0293) centre (33.7465, -24.791) ccw
  arc A53 (33.5063, -24.5833) -> (34.7366, -23.0842) centre (5.08, 0) ccw
  arc A54 (35.18, -23.027) -> (34.7366, -23.0842) centre (34.9872, -23.2792) ccw
  line L26 (35.18, -23.027) -> (35.4113, -23.2039)
  spline S26 degree 5 poles (35.4113, -23.2039) (35.423, -23.2128) (35.4466, -23.2304) (35.4826, -23.256) (35.5316, -23.2884) (35.5944, -23.3268) (35.6583, -23.3636) (35.7228, -23.3994) (35.7877, -23.4347) (35.8529, -23.4696) (35.9182, -23.5042) (35.9839, -23.5382) (36.0501, -23.5716) (36.1167, -23.6042) (36.1838, -23.636) (36.2513, -23.6671) (36.3192, -23.6976) (36.3875, -23.7275) (36.456, -23.757) (36.5247, -23.7861) (36.5937, -23.8147) (36.663, -23.8429) (36.7325, -23.8706) (36.8024, -23.8977) (36.8724, -23.9244) (36.9428, -23.9507) (37.0134, -23.9765) (37.0842, -24.0018) (37.1553, -24.0268) (37.2265, -24.0513) (37.298, -24.0754) (37.3697, -24.0992) (37.4416, -24.1225) (37.5137, -24.1455) (37.586, -24.168) (37.6585, -24.1902) (37.7311, -24.2119) (37.804, -24.2333) (37.8771, -24.2544) (37.9503, -24.275) (38.0237, -24.2953) (38.0973, -24.3153) (38.171, -24.3348) (38.2449, -24.3541) (38.319, -24.3729) (38.3933, -24.3915) (38.4677, -24.4096) (38.5422, -24.4275) (38.6169, -24.445) (38.6918, -24.4621) (38.7668, -24.4789) (38.8419, -24.4954) (38.9172, -24.5116) (38.9926, -24.5274) (39.0682, -24.5429) (39.1439, -24.5581) (39.2198, -24.573) (39.2957, -24.5875) (39.3718, -24.6017) (39.4481, -24.6156) (39.5244, -24.6292) (39.6009, -24.6425) (39.6775, -24.6555) (39.7543, -24.6682) (39.8311, -24.6805) (39.9081, -24.6926) (39.9852, -24.7043) (40.0624, -24.7157) (40.1397, -24.7269) (40.2171, -24.7377) (40.2946, -24.7483) (40.3567, -24.7565) (40.4034, -24.7625) (40.4345, -24.7664) (40.45, -24.7684) knots 0 0 0 0 0 0 0.01428571 0.02857143 0.04285714 0.05714286 0.07142857 0.08571429 0.1 0.11428571 0.12857143 0.14285714 0.15714286 0.17142857 0.18571429 0.2 0.21428571 0.22857143 0.24285714 0.25714286 0.27142857 0.28571429 0.3 0.31428571 0.32857143 0.34285714 0.35714286 0.37142857 0.38571429 0.4 0.41428571 0.42857143 0.44285714 0.45714286 0.47142857 0.48571429 0.5 0.51428571 0.52857143 0.54285714 0.55714286 0.57142857 0.58571429 0.6 0.61428571 0.62857143 0.64285714 0.65714286 0.67142857 0.68571429 0.7 0.71428571 0.72857143 0.74285714 0.75714286 0.77142857 0.78571429 0.8 0.81428571 0.82857143 0.84285714 0.85714286 0.87142857 0.88571429 0.9 0.91428571 0.92857143 0.94285714 0.95714286 0.97142857 0.98571429 1 1 1 1 1 1
  arc A55 (40.45, -24.7684) -> (41.4985, -23.1992) centre (5.08, 0) ccw
  spline S27 degree 5 poles (41.4985, -23.1992) (41.4908, -23.1856) (41.4752, -23.1583) (41.4518, -23.1176) (41.4205, -23.0633) (41.3811, -22.9957) (41.3414, -22.9283) (41.3015, -22.8612) (41.2614, -22.7942) (41.2211, -22.7275) (41.1805, -22.661) (41.1397, -22.5948) (41.0986, -22.5287) (41.0573, -22.4629) (41.0158, -22.3973) (40.974, -22.332) (40.932, -22.2669) (40.8897, -22.202) (40.8472, -22.1374) (40.8044, -22.073) (40.7614, -22.0088) (40.7182, -21.945) (40.6747, -21.8813) (40.631, -21.818) (40.587, -21.7548) (40.5427, -21.692) (40.4982, -21.6294) (40.4535, -21.5671) (40.4085, -21.505) (40.3632, -21.4432) (40.3177, -21.3817) (40.2719, -21.3205) (40.2259, -21.2596) (40.1795, -21.1989) (40.133, -21.1386) (40.0861, -21.0785) (40.039, -21.0188) (39.9916, -20.9594) (39.944, -20.9002) (39.896, -20.8414) (39.8478, -20.7829) (39.7993, -20.7247) (39.7506, -20.6669) (39.7015, -20.6094) (39.6521, -20.5523) (39.6025, -20.4955) (39.5525, -20.439) (39.5023, -20.383) (39.4517, -20.3272) (39.4009, -20.2719) (39.3498, -20.2169) (39.2983, -20.1624) (39.2464, -20.1083) (39.1942, -20.0546) (39.1417, -20.0014) (39.0889, -19.9486) (39.0357, -19.8962) (38.9822, -19.8442) (38.9285, -19.7926) (38.8743, -19.7415) (38.8197, -19.691) (38.7647, -19.6412) (38.7091, -19.5921) (38.6529, -19.5438) (38.5963, -19.4962) (38.5394, -19.449) (38.4822, -19.4022) (38.4248, -19.3557) (38.367, -19.3098) (38.3085, -19.2649) (38.249, -19.2215) (38.2003, -19.1886) (38.1629, -19.1652) (38.1376, -19.1501) (38.1249, -19.1428) knots -1 -1 -1 -1 -1 -1 -0.98571429 -0.97142857 -0.95714286 -0.94285714 -0.92857143 -0.91428571 -0.9 -0.88571429 -0.87142857 -0.85714286 -0.84285714 -0.82857143 -0.81428571 -0.8 -0.78571429 -0.77142857 -0.75714286 -0.74285714 -0.72857143 -0.71428571 -0.7 -0.68571429 -0.67142857 -0.65714286 -0.64285714 -0.62857143 -0.61428571 -0.6 -0.58571429 -0.57142857 -0.55714286 -0.54285714 -0.52857143 -0.51428571 -0.5 -0.48571429 -0.47142857 -0.45714286 -0.44285714 -0.42857143 -0.41428571 -0.4 -0.38571429 -0.37142857 -0.35714286 -0.34285714 -0.32857143 -0.31428571 -0.3 -0.28571429 -0.27142857 -0.25714286 -0.24285714 -0.22857143 -0.21428571 -0.2 -0.18571429 -0.17142857 -0.15714286 -0.14285714 -0.12857143 -0.11428571 -0.1 -0.08571429 -0.07142857 -0.05714286 -0.04285714 -0.02857143 -0.01428571 0 0 0 0 0 0
  line L27 (38.1249, -19.1428) -> (37.8729, -18.9968)
  arc A56 (37.7561, -18.5652) -> (37.8729, -18.9968) centre (38.0322, -18.7221) ccw
  arc A57 (37.7561, -18.5652) -> (38.6703, -16.8549) centre (5.08, 0) ccw
  arc A58 (39.094, -16.7123) -> (38.6703, -16.8549) centre (38.9541, -16.9973) ccw
  line L28 (39.094, -16.7123) -> (39.3554, -16.8407)
  spline S28 degree 5 poles (39.3554, -16.8407) (39.3686, -16.8471) (39.3951, -16.8598) (39.4354, -16.8779) (39.4898, -16.9001) (39.5589, -16.9255) (39.6288, -16.9492) (39.699, -16.9717) (39.7696, -16.9936) (39.8403, -17.0152) (39.9111, -17.0363) (39.9822, -17.0569) (40.0536, -17.0767) (40.1253, -17.0957) (40.1973, -17.1138) (40.2696, -17.1311) (40.3422, -17.1478) (40.4149, -17.1638) (40.4879, -17.1794) (40.561, -17.1945) (40.6342, -17.2091) (40.7077, -17.2232) (40.7813, -17.2368) (40.855, -17.2498) (40.929, -17.2623) (41.0031, -17.2744) (41.0774, -17.2859) (41.1518, -17.2969) (41.2263, -17.3075) (41.301, -17.3177) (41.3758, -17.3274) (41.4508, -17.3367) (41.5258, -17.3456) (41.601, -17.354) (41.6763, -17.362) (41.7517, -17.3696) (41.8273, -17.3768) (41.9029, -17.3836) (41.9787, -17.3899) (42.0545, -17.3959) (42.1305, -17.4015) (42.2065, -17.4067) (42.2827, -17.4115) (42.3589, -17.416) (42.4353, -17.42) (42.5117, -17.4237) (42.5882, -17.427) (42.6648, -17.43) (42.7415, -17.4325) (42.8183, -17.4348) (42.8951, -17.4366) (42.972, -17.4381) (43.049, -17.4393) (43.1261, -17.4401) (43.2032, -17.4406) (43.2804, -17.4407) (43.3577, -17.4405) (43.4351, -17.4399) (43.5125, -17.439) (43.59, -17.4378) (43.6675, -17.4362) (43.7451, -17.4343) (43.8228, -17.4321) (43.9005, -17.4295) (43.9783, -17.4267) (44.0561, -17.4235) (44.134, -17.42) (44.212, -17.4161) (44.29, -17.412) (44.368, -17.4075) (44.4461, -17.4027) (44.5086, -17.3986) (44.5556, -17.3954) (44.5868, -17.3932) (44.6025, -17.3921) knots 0 0 0 0 0 0 0.01428571 0.02857143 0.04285714 0.05714286 0.07142857 0.08571429 0.1 0.11428571 0.12857143 0.14285714 0.15714286 0.17142857 0.18571429 0.2 0.21428571 0.22857143 0.24285714 0.25714286 0.27142857 0.28571429 0.3 0.31428571 0.32857143 0.34285714 0.35714286 0.37142857 0.38571429 0.4 0.41428571 0.42857143 0.44285714 0.45714286 0.47142857 0.48571429 0.5 0.51428571 0.52857143 0.54285714 0.55714286 0.57142857 0.58571429 0.6 0.61428571 0.62857143 0.64285714 0.65714286 0.67142857 0.68571429 0.7 0.71428571 0.72857143 0.74285714 0.75714286 0.77142857 0.78571429 0.8 0.81428571 0.82857143 0.84285714 0.85714286 0.87142857 0.88571429 0.9 0.91428571 0.92857143 0.94285714 0.95714286 0.97142857 0.98571429 1 1 1 1 1 1
  arc A59 (44.6025, -17.3921) -> (45.3247, -15.6485) centre (5.08, 0) ccw
  spline S29 degree 5 poles (45.3247, -15.6485) (45.3144, -15.6367) (45.2939, -15.613) (45.263, -15.5776) (45.2216, -15.5305) (45.1698, -15.4719) (45.1178, -15.4135) (45.0655, -15.3554) (45.0131, -15.2976) (44.9606, -15.24) (44.9078, -15.1827) (44.8548, -15.1257) (44.8017, -15.0689) (44.7483, -15.0125) (44.6948, -14.9562) (44.641, -14.9003) (44.5871, -14.8446) (44.533, -14.7893) (44.4787, -14.7342) (44.4242, -14.6794) (44.3695, -14.6248) (44.3147, -14.5706) (44.2596, -14.5167) (44.2043, -14.4631) (44.1489, -14.4098) (44.0932, -14.3567) (44.0374, -14.304) (43.9813, -14.2516) (43.9251, -14.1996) (43.8686, -14.1478) (43.812, -14.0964) (43.7551, -14.0452) (43.6981, -13.9945) (43.6408, -13.944) (43.5834, -13.8939) (43.5257, -13.8442) (43.4678, -13.7948) (43.4098, -13.7457) (43.3515, -13.697) (43.293, -13.6487) (43.2343, -13.6007) (43.1754, -13.5531) (43.1163, -13.5059) (43.0569, -13.4591) (42.9974, -13.4127) (42.9376, -13.3667) (42.8776, -13.3211) (42.8174, -13.2758) (42.7569, -13.231) (42.6963, -13.1867) (42.6354, -13.1427) (42.5742, -13.0993) (42.5129, -13.0564) (42.4512, -13.0139) (42.3893, -12.972) (42.3272, -12.9305) (42.2648, -12.8895) (42.2022, -12.8489) (42.1394, -12.8088) (42.0764, -12.7693) (42.013, -12.7304) (41.9492, -12.6922) (41.8851, -12.655) (41.8206, -12.6185) (41.7558, -12.5828) (41.6908, -12.5477) (41.6256, -12.5129) (41.5602, -12.4786) (41.4945, -12.4448) (41.4284, -12.4121) (41.3616, -12.3812) (41.3074, -12.3585) (41.2662, -12.3428) (41.2384, -12.333) (41.2245, -12.3282) knots -1 -1 -1 -1 -1 -1 -0.98571429 -0.97142857 -0.95714286 -0.94285714 -0.92857143 -0.91428571 -0.9 -0.88571429 -0.87142857 -0.85714286 -0.84285714 -0.82857143 -0.81428571 -0.8 -0.78571429 -0.77142857 -0.75714286 -0.74285714 -0.72857143 -0.71428571 -0.7 -0.68571429 -0.67142857 -0.65714286 -0.64285714 -0.62857143 -0.61428571 -0.6 -0.58571429 -0.57142857 -0.55714286 -0.54285714 -0.52857143 -0.51428571 -0.5 -0.48571429 -0.47142857 -0.45714286 -0.44285714 -0.42857143 -0.41428571 -0.4 -0.38571429 -0.37142857 -0.35714286 -0.34285714 -0.32857143 -0.31428571 -0.3 -0.28571429 -0.27142857 -0.25714286 -0.24285714 -0.22857143 -0.21428571 -0.2 -0.18571429 -0.17142857 -0.15714286 -0.14285714 -0.12857143 -0.11428571 -0.1 -0.08571429 -0.07142857 -0.05714286 -0.04285714 -0.02857143 -0.01428571 0 0 0 0 0 0
  line L29 (41.2245, -12.3282) -> (40.9489, -12.2341)
  arc A60 (40.7501, -11.8337) -> (40.9489, -12.2341) centre (41.0515, -11.9337) ccw
  arc A61 (40.7501, -11.8337) -> (41.3131, -9.9779) centre (5.08, 0) ccw
  arc A62 (41.7008, -9.7554) -> (41.3131, -9.9779) centre (41.6192, -10.0622) ccw
  line L30 (41.7008, -9.7554) -> (41.9822, -9.8303)
  spline S30 degree 5 poles (41.9822, -9.8303) (41.9964, -9.8341) (42.025, -9.8413) (42.068, -9.8512) (42.1257, -9.8624) (42.1984, -9.8738) (42.2715, -9.8834) (42.3449, -9.8917) (42.4183, -9.8995) (42.4919, -9.9069) (42.5655, -9.9138) (42.6392, -9.9201) (42.7131, -9.9256) (42.7871, -9.9302) (42.8613, -9.934) (42.9356, -9.9368) (43.01, -9.939) (43.0845, -9.9405) (43.1591, -9.9416) (43.2337, -9.9421) (43.3084, -9.9421) (43.3832, -9.9416) (43.458, -9.9406) (43.5329, -9.939) (43.6079, -9.9369) (43.6829, -9.9342) (43.758, -9.931) (43.8331, -9.9273) (43.9083, -9.9232) (43.9836, -9.9186) (44.0588, -9.9135) (44.1341, -9.908) (44.2095, -9.9021) (44.2849, -9.8957) (44.3603, -9.8888) (44.4358, -9.8816) (44.5112, -9.8739) (44.5868, -9.8657) (44.6623, -9.8572) (44.7379, -9.8483) (44.8134, -9.8389) (44.889, -9.8292) (44.9647, -9.8191) (45.0403, -9.8086) (45.116, -9.7976) (45.1916, -9.7863) (45.2673, -9.7747) (45.343, -9.7626) (45.4188, -9.7502) (45.4945, -9.7374) (45.5702, -9.7242) (45.6459, -9.7107) (45.7217, -9.6968) (45.7974, -9.6826) (45.8732, -9.668) (45.9489, -9.653) (46.0247, -9.6377) (46.1005, -9.6221) (46.1762, -9.6061) (46.252, -9.5898) (46.3277, -9.5731) (46.4035, -9.5561) (46.4792, -9.5388) (46.5549, -9.5211) (46.6307, -9.5031) (46.7064, -9.4848) (46.7821, -9.4662) (46.8578, -9.4472) (46.9335, -9.4279) (47.0092, -9.4083) (47.0848, -9.3884) (47.1453, -9.3722) (47.1907, -9.3599) (47.221, -9.3516) (47.2361, -9.3475) knots 0 0 0 0 0 0 0.01428571 0.02857143 0.04285714 0.05714286 0.07142857 0.08571429 0.1 0.11428571 0.12857143 0.14285714 0.15714286 0.17142857 0.18571429 0.2 0.21428571 0.22857143 0.24285714 0.25714286 0.27142857 0.28571429 0.3 0.31428571 0.32857143 0.34285714 0.35714286 0.37142857 0.38571429 0.4 0.41428571 0.42857143 0.44285714 0.45714286 0.47142857 0.48571429 0.5 0.51428571 0.52857143 0.54285714 0.55714286 0.57142857 0.58571429 0.6 0.61428571 0.62857143 0.64285714 0.65714286 0.67142857 0.68571429 0.7 0.71428571 0.72857143 0.74285714 0.75714286 0.77142857 0.78571429 0.8 0.81428571 0.82857143 0.84285714 0.85714286 0.87142857 0.88571429 0.9 0.91428571 0.92857143 0.94285714 0.95714286 0.97142857 0.98571429 1 1 1 1 1 1
  arc A63 (47.2361, -9.3475) -> (47.6043, -7.4965) centre (5.08, 0) ccw
  spline S31 degree 5 poles (47.6043, -7.4965) (47.5919, -7.4869) (47.5671, -7.4677) (47.5299, -7.4389) (47.4802, -7.4008) (47.4179, -7.3535) (47.3555, -7.3064) (47.2929, -7.2596) (47.2303, -7.2131) (47.1674, -7.1669) (47.1045, -7.121) (47.0414, -7.0754) (46.9782, -7.0301) (46.9149, -6.9851) (46.8514, -6.9404) (46.7878, -6.896) (46.7241, -6.8519) (46.6602, -6.8082) (46.5962, -6.7647) (46.532, -6.7216) (46.4678, -6.6788) (46.4034, -6.6364) (46.3388, -6.5942) (46.2742, -6.5524) (46.2094, -6.5109) (46.1444, -6.4698) (46.0794, -6.429) (46.0142, -6.3885) (45.9489, -6.3484) (45.8834, -6.3087) (45.8178, -6.2693) (45.7521, -6.2302) (45.6862, -6.1916) (45.6202, -6.1533) (45.5541, -6.1153) (45.4879, -6.0778) (45.4215, -6.0406) (45.3549, -6.0038) (45.2883, -5.9674) (45.2215, -5.9314) (45.1546, -5.8958) (45.0875, -5.8606) (45.0203, -5.8259) (44.953, -5.7916) (44.8855, -5.7577) (44.8179, -5.7242) (44.7501, -5.6912) (44.6823, -5.6586) (44.6142, -5.6264) (44.5461, -5.5947) (44.4778, -5.5635) (44.4093, -5.5328) (44.3408, -5.5027) (44.272, -5.4731) (44.2031, -5.444) (44.1341, -5.4155) (44.0649, -5.3874) (43.9956, -5.3598) (43.9262, -5.3328) (43.8566, -5.3063) (43.7869, -5.2805) (43.7169, -5.2555) (43.6468, -5.2315) (43.5764, -5.2083) (43.5059, -5.186) (43.4353, -5.1642) (43.3645, -5.1428) (43.2936, -5.1219) (43.2227, -5.1016) (43.1515, -5.0824) (43.0799, -5.0651) (43.0223, -5.0534) (42.9788, -5.0461) (42.9497, -5.0418) (42.9351, -5.0399) knots -1 -1 -1 -1 -1 -1 -0.98571429 -0.97142857 -0.95714286 -0.94285714 -0.92857143 -0.91428571 -0.9 -0.88571429 -0.87142857 -0.85714286 -0.84285714 -0.82857143 -0.81428571 -0.8 -0.78571429 -0.77142857 -0.75714286 -0.74285714 -0.72857143 -0.71428571 -0.7 -0.68571429 -0.67142857 -0.65714286 -0.64285714 -0.62857143 -0.61428571 -0.6 -0.58571429 -0.57142857 -0.55714286 -0.54285714 -0.52857143 -0.51428571 -0.5 -0.48571429 -0.47142857 -0.45714286 -0.44285714 -0.42857143 -0.41428571 -0.4 -0.38571429 -0.37142857 -0.35714286 -0.34285714 -0.32857143 -0.31428571 -0.3 -0.28571429 -0.27142857 -0.25714286 -0.24285714 -0.22857143 -0.21428571 -0.2 -0.18571429 -0.17142857 -0.15714286 -0.14285714 -0.12857143 -0.11428571 -0.1 -0.08571429 -0.07142857 -0.05714286 -0.04285714 -0.02857143 -0.01428571 0 0 0 0 0 0
  line L31 (42.9351, -5.0399) -> (42.6465, -5.0014)
  arc A64 (42.3734, -4.6474) -> (42.6465, -5.0014) centre (42.6884, -4.6867) ccw
  arc A65 (42.3734, -4.6474) -> (42.5635, -2.7175) centre (5.08, 0) ccw
  arc A66 (42.9004, -2.4236) -> (42.5635, -2.7175) centre (42.8801, -2.7404) ccw
  line L32 (42.9004, -2.4236) -> (43.1909, -2.4421)